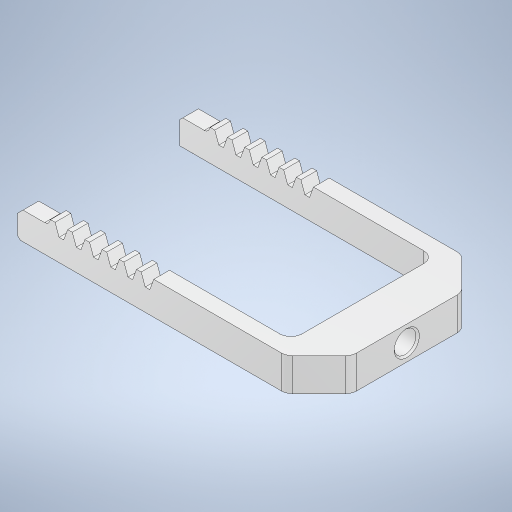
# Autodesk Inventor part: Rack
Saved by Autodesk Inventor 2023.4 (Build 274418000, 418)
## iProperties
Created: 2024-01-11
Part Number: Rack
Material: Aluminum 6061
Document SubType Name: Modeling
Designer: Nathan Cai
Mass: 18.3268 g
Surface Area: 57.6486 cm^2
Volume: 6.78771 cm^3
Density: 2.7 g/cm^3
Appearance: Aluminum - Flat
Author: Nathan Cai
Autodesk Inventor part; units mm, degrees
ref_plane "YZ Plane" through (0, 0, 0) normal (1, 0, 0) x (0, 1, 0)
ref_plane "XZ Plane" through (0, 0, 0) normal (0, 1, 0) x (-1, 0, 0)
ref_plane "XY Plane" through (0, 0, 0) normal (0, 0, 1) x (1, 0, 0)
sketch "Sketch1" plane through (0, 0, 0) normal (0, 1, 0) x (-1, 0, 0)
  line L0 (37.3062, 20.85) -> (-37.3063, 20.85)
  line L1 (-37.3063, 20.85) -> (-37.3062, -20.85)
  line L2 (-37.3062, -20.85) -> (37.3063, -20.85)
  line L3 (37.3063, -20.85) -> (37.3062, 20.85)
  line L4 (37.3062, 20.85) -> (-37.3062, -20.85) construction
  line L5 (-37.3063, 20.85) -> (37.3063, -20.85) construction
  line L6 (0, 0) -> (-37.3062, 0) construction
  line L7 (37.3063, 25.4) -> (-50.0062, 25.4)
  line L8 (-50.0062, 25.4) -> (-50.0062, -25.4)
  line L9 (-50.0062, -25.4) -> (37.3063, -25.4)
  line L10 (37.3063, -25.4) -> (37.3063, 25.4)
  line L11 (37.3063, 25.4) -> (-50.0062, -25.4) construction
  line L12 (-50.0062, 25.4) -> (37.3063, -25.4) construction
  point P0 (-6.35, 0)
  point P1 (37.3063, 20.85)
  dimension "d0" = 74.6125
  dimension "d1" = 41.7
  dimension "d3" = 12.7
  dimension "d198" = 50.8
  constraints: 26 end point, 5 midpoint, 4 parallel, 2 horizontal, 2 perpendicular, 2 point on line
  measures "d0" distance of L2.end L1.end
  measures "d1" distance of L1.end L0.end
  measures "d3" distance between parallel lines of L1 L8
  measures "d198" distance between parallel lines of L7 L9
extrude "Extrusion1" add sketch "Sketch1" along normal blind 9.525 contours L0 L1 L2 L10 L9 L8 L7
chamfer "Chamfer1" distance 9.525 angle 45 2 edges at (50.0062, 4.7625, 25.4) (50.0062, 4.7625, -25.4)
fillet "Fillet1" radius 3.175 4 edges at (40.4812, 4.7625, -25.4) (50.0062, 4.7625, -15.875) (50.0062, 4.7625, 15.875) (40.4812, 4.7625, 25.4)
fillet "Fillet4" radius 3.175 2 edges at (37.3062, 4.7625, -20.85) (37.3063, 4.7625, 20.85)
sketch "Sketch5" plane through (-37.3063, 0, -25.4) normal (0, 0, -1) x (-1, 0, 0)
  line L0 (0, 0) -> (0, 9.525) projected
  line L1 (0, 9.525) -> (-76.4724, 9.525) projected
  line L2 (-10.8754, 9.525) -> (-12.031, 6.35)
  line L3 (-12.031, 6.35) -> (-13.369, 6.35)
  line L4 (-13.369, 6.35) -> (-14.5246, 9.525)
  line L5 (-25.4, 9.525) -> (-25.4, 6.35) construction
  line L6 (0, 9.525) -> (0, 6.35) construction
  line L7 (-12.7, 9.525) -> (-12.7, 6.35) construction
  line L8 (-25.4, 7.9375) -> (0, 7.9375) construction
  line L9 (-15.8627, 9.525) -> (-17.0183, 6.35)
  line L10 (-17.0183, 6.35) -> (-18.3563, 6.35)
  line L11 (-18.3563, 6.35) -> (-19.5119, 9.525)
  line L12 (-17.6873, 9.525) -> (-17.6873, 6.35) construction
  line L13 (-20.8499, 9.525) -> (-22.0055, 6.35)
  line L14 (-22.0055, 6.35) -> (-23.3436, 6.35)
  line L15 (-23.3436, 6.35) -> (-24.4992, 9.525)
  line L16 (-22.6746, 9.525) -> (-22.6746, 6.35) construction
  line L17 (-25.8372, 9.525) -> (-26.9928, 6.35)
  line L18 (-26.9928, 6.35) -> (-28.3309, 6.35)
  line L19 (-28.3309, 6.35) -> (-29.4865, 9.525)
  line L20 (-27.6618, 9.525) -> (-27.6618, 6.35) construction
  line L21 (-30.8245, 9.525) -> (-31.9801, 6.35)
  line L22 (-31.9801, 6.35) -> (-33.3181, 6.35)
  line L23 (-33.3181, 6.35) -> (-34.4737, 9.525)
  line L24 (-32.6491, 9.525) -> (-32.6491, 6.35) construction
  line L25 (-35.8118, 9.525) -> (-36.9674, 6.35)
  line L26 (-36.9674, 6.35) -> (-38.3054, 6.35)
  line L27 (-38.3054, 6.35) -> (-39.461, 9.525)
  line L28 (-37.6364, 9.525) -> (-37.6364, 6.35) construction
  line L29 (-12.031, 6.35) -> (0, 6.35)
  line L30 (-5.8881, 9.525) -> (-7.0437, 6.35)
  line L31 (-8.3817, 6.35) -> (-9.5373, 9.525)
  line L32 (-8.9595, 7.9375) -> (0, 7.9375)
  arc A0 (-8.3817, 6.35) -> (-7.0437, 6.35) centre (-7.7127, 6.5935) ccw
  arc A1 (-13.369, 6.35) -> (-12.031, 6.35) centre (-12.7, 6.5935) ccw
  arc A2 (-18.3563, 6.35) -> (-17.0183, 6.35) centre (-17.6873, 6.5935) ccw
  arc A3 (-23.3436, 6.35) -> (-22.0055, 6.35) centre (-22.6746, 6.5935) ccw
  arc A4 (-28.3309, 6.35) -> (-26.9928, 6.35) centre (-27.6618, 6.5935) ccw
  arc A5 (-33.3181, 6.35) -> (-31.9801, 6.35) centre (-32.6491, 6.5935) ccw
  arc A6 (-38.3054, 6.35) -> (-36.9674, 6.35) centre (-37.6364, 6.5935) ccw
  point P0 (-37.3062, 0)
  point P1 (-13.9468, 7.9375)
  point P2 (-11.4532, 7.9375)
  point P3 (-11.4532, 7.9375)
  point P4 (-16.4405, 7.9375)
  point P5 (-16.4405, 7.9375)
  point P6 (-4.9873, 6.35)
  point P7 (-30.3873, 6.35)
  point P8 (-18.9341, 7.9375)
  point P9 (-21.4277, 7.9375)
  point P10 (-21.4277, 7.9375)
  point P11 (-9.9746, 6.35)
  point P12 (-35.3746, 6.35)
  point P13 (-23.9214, 7.9375)
  point P14 (-26.415, 7.9375)
  point P15 (-26.415, 7.9375)
  point P16 (-14.9618, 6.35)
  point P17 (-40.3618, 6.35)
  point P18 (-28.9087, 7.9375)
  point P19 (-31.4023, 7.9375)
  point P20 (-31.4023, 7.9375)
  point P21 (-19.9491, 6.35)
  point P22 (-45.3491, 6.35)
  point P23 (-33.8959, 7.9375)
  point P24 (-36.3896, 7.9375)
  point P25 (-36.3896, 7.9375)
  point P26 (-24.9364, 6.35)
  point P27 (-50.3364, 6.35)
  point P28 (-38.8832, 7.9375)
  point P29 (-24.4992, 9.525)
  point P30 (-6.4659, 7.9375)
  point P31 (-6.4659, 7.9375)
  point P32 (0, 7.9375)
  dimension "d68" = 3.175
  dimension "d70" = 70
  dimension "d71" = 2.4936
  dimension "d74" = 4.9873
  dimension "d79" = 12.7
  dimension "d82" = 4.9873
  dimension "d175" = 4.9873
  constraints: 62 end point, 20 point on line, 18 midpoint, 14 point on circle, 7 centre point, 5 horizontal, 2 tangent, 1 collinear, 1 vertical, 110 other
  measures "d68" distance from line of L1 L6.end
  measures "d70" angle of L3 L2
  measures "d71" distance of point (-11.453, 7.938) point (-13.947, 7.938)
  measures "d74" distance of L2.start L9.start
  measures "d79" distance between parallel lines of L0 L7
  measures "d82" distance of L2.start L30.start
  measures "d175" distance of A0.centre A1.centre
extrude "Extrusion8" cut sketch "Sketch5" against normal through all contours L32 L30 L1 L0 | L32 L31 L1 L30 | L3 L4 L1 L2 | L9 L10 L11 L1 | L13 L14 L15 L1 | L17 L18 L19 L1 | L21 L22 L23 L1 | L25 L26 L27 L1
fillet "Fillet5" radius 1.5875 2 edges at (-28.3467, 7.9375, -23.125) (-28.3467, 7.9375, 23.125)
chamfer "Chamfer3" distance 1.5875 angle 45 2 edges at (-37.3063, 7.9375, -23.125) (-37.3062, 7.9375, 23.125)
chamfer "Chamfer4" distance 0.7937 angle 45 2 edges at (-37.3063, 0, -23.125) (-37.3063, 0, 23.125)
ref_plane "Work Plane3" through (0, 4.7625, 0) normal (0, 1, 0) x (1, 0, 0)
sketch "Sketch14" plane through (50.0062, 0, 14.5599) normal (1, 0, 0) x (0, 0, -1)
  line L0 (14.5599, 0) -> (14.5599, 9.525) construction
  line L1 (32.2349, 9.525) -> (-3.1151, 9.525) projected
  circle A0 centre (14.5599, 4.7625) radius 3.175
  dimension "d199" = 6.35
  constraints: 2 end point, 2 midpoint, 1 centre point
  measures "d199" diameter of A0
extrude "Extrusion19" cut sketch "Sketch14" against normal through all
chamfer "Chamfer12" distance 0.5 angle 45 2 edges at (50.0062, 4.7625, 3.175) (37.3063, 4.7625, 3.175)
chamfer "Chamfer8" distance 0.7937 angle 45 2 edges at (-37.3063, 3.5719, -20.85) (-37.3063, 3.5719, 20.85)
chamfer "Chamfer11" distance 0.5 angle 45 5 edges at (-1.1906, 0, -20.85) (36.3763, 0, -19.9201) (37.3062, 0, 0) (36.3763, 0, 19.9201) (-1.1906, 0, 20.85)
equation "\"d71\" = 0.5 * d69"
equation "\"d74\" = 1.5708 * d68"
equation "\"d82\" = d74"
equation "\"d69\" = 1.5708 * d68"
body "Solid1"
